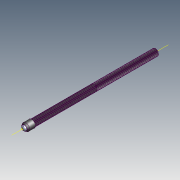
# Autodesk Inventor part: T-NA08A50-S_Shaft
Saved by Autodesk Inventor 2015 SP1 (Build 190203100, 203)
## iProperties
Created: 2014-09-03
Part Number: T-NA08A50-S_Shaft
Material: Generic
Document SubType Name: Modeling
Designer: arnoldj
Density: 1 g/cm^3
Appearance: Default
Translation Standard: STEP AP214IS
FileName: C:\_WORKSPACE\DATA\Imported Components\T-NA08x25 rev2\T-NA08x25_Shaft.stp
PreProcessor: Autodesk Inventor 2012
PostProcessor: Build: 219, Release: 2012 SP2 - Date: Fri 04/27/2012
Sent Units: millimeter
Uncertainty: 0.01
Revision Number: 0
Autodesk Inventor part; units mm, degrees
ref_plane "YZ Plane" through (0, 0, 0) normal (1, 0, 0) x (0, 1, 0)
ref_plane "XZ Plane" through (0, 0, 0) normal (0, 1, 0) x (-1, 0, 0)
ref_plane "XY Plane" through (0, 0, 0) normal (0, 0, 1) x (1, 0, 0)
surface "Composite1"
sketch "Sketch1" plane through (-12.6252, -7.613, 24.9968) normal (0, 0, 1) x (0.8491307, 0.5281828, 0)
  line L0 (0.7285, 0.1548) -> (0.9799, 0.501) projected
  line L1 (1.0926, 0.0573) -> (1.0479, 0.4828) projected
  line L2 (1.4388, 0.3088) -> (1.0926, 0.0573) projected
  line L3 (1.4978, 0.2704) -> (1.4088, -0.1481) projected
  line L4 (1.8157, -0.0159) -> (1.4088, -0.1481) projected
  line L5 (1.6461, -0.4411) -> (1.86, -0.0705) projected
  line L6 (1.6461, -0.4411) -> (2.0739, -0.4411) projected
  line L7 (1.7812, -0.793) -> (2.0991, -0.5067) projected
  line L8 (2.1881, -0.9252) -> (1.7812, -0.793) projected
  line L9 (2.1918, -0.9955) -> (1.8009, -1.1695) projected
  line L10 (2.147, -1.421) -> (1.8009, -1.1695) projected
  line L11 (1.7033, -1.5337) -> (2.1288, -1.489) projected
  line L12 (1.9548, -1.8798) -> (1.7033, -1.5337) projected
  line L13 (1.498, -1.8499) -> (1.9165, -1.9388) projected
  line L14 (1.6302, -2.2568) -> (1.498, -1.8499) projected
  line L15 (1.205, -2.0871) -> (1.5755, -2.3011) projected
  line L16 (1.205, -2.515) -> (1.205, -2.0871) projected
  line L17 (0.853, -2.2222) -> (1.1393, -2.5402) projected
  line L18 (0.7208, -2.6292) -> (0.853, -2.2222) projected
  line L19 (0.4765, -2.242) -> (0.6506, -2.6328) projected
  line L20 (0.2251, -2.5881) -> (0.4765, -2.242) projected
  line L21 (0.1124, -2.1444) -> (0.1571, -2.5699) projected
  line L22 (-0.2338, -2.3959) -> (0.1124, -2.1444) projected
  line L23 (-0.2038, -1.9391) -> (-0.2928, -2.3576) projected
  line L24 (-0.6107, -2.0713) -> (-0.2038, -1.9391) projected
  line L25 (-0.655, -2.0166) -> (-0.4411, -1.6461) projected
  line L26 (-0.4411, -1.6461) -> (-0.8689, -1.6461) projected
  line L27 (-0.5762, -1.2941) -> (-0.8941, -1.5804) projected
  line L28 (-0.5762, -1.2941) -> (-0.9831, -1.1619) projected
  line L29 (-0.5959, -0.9176) -> (-0.9868, -1.0916) projected
  line L30 (-0.4983, -0.5534) -> (-0.9238, -0.5982) projected
  line L31 (-0.942, -0.6661) -> (-0.5959, -0.9176) projected
  line L32 (-0.7498, -0.2073) -> (-0.4983, -0.5534) projected
  line L33 (-0.293, -0.2373) -> (-0.7115, -0.1483) projected
  line L34 (-0.4252, 0.1697) -> (-0.293, -0.2373) projected
  line L35 (0, 0) -> (-0.3705, 0.2139) projected
  line L36 (0, 0.4279) -> (0, 0) projected
  line L37 (0.352, 0.1351) -> (0.0657, 0.4531) projected
  line L38 (0.352, 0.1351) -> (0.4842, 0.542) projected
  line L39 (0.7285, 0.1548) -> (0.5544, 0.5457) projected
  arc A0 (1.86, -0.0705) -> (1.8157, -0.0159) centre (0.6025, -1.0436) ccw projected
  arc A1 (1.4978, 0.2704) -> (1.4388, 0.3088) centre (0.6025, -1.0436) ccw projected
  arc A2 (1.0479, 0.4828) -> (0.9799, 0.501) centre (0.6025, -1.0436) ccw projected
  arc A3 (0.5544, 0.5457) -> (0.4842, 0.542) centre (0.6025, -1.0436) ccw projected
  arc A4 (0.0657, 0.4531) -> (0, 0.4279) centre (0.6025, -1.0436) ccw projected
  arc A5 (-0.3705, 0.2139) -> (-0.4252, 0.1697) centre (0.6025, -1.0436) ccw projected
  arc A6 (-0.7115, -0.1483) -> (-0.7498, -0.2073) centre (0.6025, -1.0436) ccw projected
  arc A7 (-0.9238, -0.5982) -> (-0.942, -0.6661) centre (0.6025, -1.0436) ccw projected
  arc A8 (-0.9868, -1.0916) -> (-0.9831, -1.1619) centre (0.6025, -1.0436) ccw projected
  arc A9 (-0.8941, -1.5804) -> (-0.8689, -1.6461) centre (0.6025, -1.0436) ccw projected
  arc A10 (-0.655, -2.0166) -> (-0.6107, -2.0713) centre (0.6025, -1.0436) ccw projected
  arc A11 (-0.2928, -2.3576) -> (-0.2338, -2.3959) centre (0.6025, -1.0436) ccw projected
  arc A12 (0.1571, -2.5699) -> (0.2251, -2.5881) centre (0.6025, -1.0436) ccw projected
  arc A13 (0.6506, -2.6328) -> (0.7208, -2.6292) centre (0.6025, -1.0436) ccw projected
  arc A14 (1.1393, -2.5402) -> (1.205, -2.515) centre (0.6025, -1.0436) ccw projected
  arc A15 (1.5755, -2.3011) -> (1.6302, -2.2568) centre (0.6025, -1.0436) ccw projected
  arc A16 (1.9165, -1.9388) -> (1.9548, -1.8798) centre (0.6025, -1.0436) ccw projected
  arc A17 (2.1288, -1.489) -> (2.147, -1.421) centre (0.6025, -1.0436) ccw projected
  arc A18 (2.1918, -0.9955) -> (2.1881, -0.9252) centre (0.6025, -1.0436) ccw projected
  arc A19 (2.0991, -0.5067) -> (2.0739, -0.4411) centre (0.6025, -1.0436) ccw projected
  point P0 (14.7415, -0.204)
extrude "Extrusion1" add sketch "Sketch1" against normal blind 30
body "Solid1"
body "Srf1"
